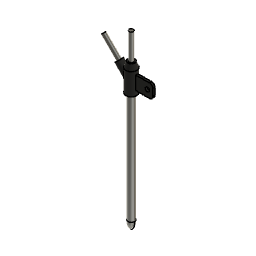
Pitot Tube Holybro (Autodesk Fusion 360 design; units mm, degrees)
Autodesk Fusion 360 part; units mm, degrees
sketch "Sketch1" plane through (0, 0, 0) normal (0, 0, 1) x (1, 0, 0)
  circle A0 centre (0, 0) radius 3.25
  dimension "d1" = 6.5
  constraint coincident A0.centre origin
  measures "d1" diameter of A0
extrude "Extrude1" add sketch "Sketch1" along normal blind 13 makes body 1
ref_plane "WorkPlane1" through (0, 0, 16.3) normal (0, 0, 1) x (1, 0, 0)
sketch "Sketch2" plane through (0, 0, 16.3) normal (0, 0, 1) x (1, 0, 0)
  circle A0 centre (0, 0) radius 2.15
  dimension "d5" = 4.3
  constraint coincident A0.centre origin
  measures "d5" diameter of A0
loft "Loft1" add profiles "Sketch2" section 1 face at (0.0595, 0.9382, 13) section 2 on bodies 1 bodies 1
sketch "Sketch3" plane through (0, 0, 16.3) normal (0, 0, 1) x (-1, 0, 0)
  circle A0 centre (0, 0) radius 2.15
  circle A1 centre (0, 0) radius 1.25
  dimension "d6" = 2.5
  constraint concentric A0 A1
  measures "d6" diameter of A1
extrude "Extrude2" add sketch "Sketch3" along normal blind 15.75 separate body contours A1 makes body 2
sketch "Sketch4" plane through (0, 0, 0) normal (0, 1, 0) x (1, 0, 0)
  line L0 (-3.25, -13) -> (3.25, -13)
  line L1 (-3.25, 0) -> (3.25, 0)
  line L2 (3.25, 0) -> (3.25, -13)
  line L3 (3.25, -3) -> (3.25, -11)
  line L4 (0, -3) -> (13.45, -3)
  line L5 (13.45, -3) -> (13.45, -11)
  line L6 (13.45, -11) -> (0, -11)
  line L7 (0, -11) -> (0, -3)
  circle A0 centre (10.25, -7) radius 1.25
  dimension "d12" = 10.2
  dimension "d13" = 3
  dimension "d14" = 8
  dimension "d15" = 4
  dimension "d16" = 3.2
  dimension "d17" = 2.5
  constraint coincident L1.end L2.start
  constraint coincident L0.end L2.end
  constraint vertical L3
  constraint coincident L2 L3.end
  constraint horizontal L4
  constraint vertical L5
  constraint horizontal L6
  constraint vertical L7
  constraint coincident origin L7
  measures "d12" distance of L1.end L5
  measures "d13" distance of L1.end L4
  measures "d14" distance of L4.end L5.end
  measures "d15" distance of L4 A0.centre
  measures "d16" distance of L5 A0.centre
  measures "d17" diameter of A0
extrude "Extrude3" add sketch "Sketch4" along normal mid plane 1.3 contours L2 L3 L4 L5 L6 bodies 2 1
fillet "Fillet1" radius 1.85 2 edges at (13.45, 0, 11) (13.45, 0, 3) on bodies 1
sketch "Sketch5" plane through (0, 0, 0) normal (0, 0, -1) x (1, 0, 0)
  circle A0 centre (0, 0) radius 3.25
  circle A1 centre (0, 0) radius 2
  dimension "d22" = 4
  constraint coincident A0.centre A1.centre
  measures "d22" diameter of A1
extrude "Extrude4" add sketch "Sketch5" along normal blind 65.7 separate body contours A1 makes body 3
sketch "Sketch6" plane through (0, 0, 0) normal (0, 1, 0) x (1, 0, 0)
  line L0 (2, 65.7) -> (-2, 65.7)
  line L1 (0, 65.7) -> (0, 70.7)
  line L2 (0, 70.7) -> (0.2, 70.7)
  spline S0 degree 5 poles (2, 65.7) (2, 65.822) (1.9982, 66.0643) (1.9904, 66.4231) (1.9681, 66.8915) (1.9135, 67.4579) (1.8222, 68.0018) (1.6848, 68.5199) (1.4938, 69.0096) (1.2482, 69.4714) (0.9504, 69.9067) (0.6731, 70.2355) (0.4445, 70.4717) (0.283, 70.6246) (0.2, 70.7) knots 0 0 0 0 0 0 0.1 0.2 0.3 0.4 0.5 0.6 0.7 0.8 0.9 1 1 1 1 1 1
  line L3 (2, 65.0687) -> (2, 66.3313)
  line L4 (2, 65.7) -> (0, 65.7)
  point P0 (1.6554, 68.5611)
  dimension "d25" = 5
  dimension "d26" = 0.2
  constraint midpoint L0 L1.start
  constraint perpendicular L0 L1
  constraint perpendicular L1 L2
  constraint coincident L0.start S0.start
  constraint midpoint L0.start L3
  constraint vertical L3
  measures "d25" distance of L1.start L1.end
  measures "d26" distance of L1.end L2.end
revolve "Revolve1" add sketch "Sketch6" angle 360 about axis through (0, 0, -65.7) along (0, 0, -1) bodies 3
ref_plane "WorkPlane2" through (0, 12.125, 0) normal (-0.707107, 0, 0.707107) x (0, 1, 0)
sketch "Sketch7" plane through (0, 12.125, 0) normal (-0.707107, 0, 0.707107) x (0, 1, 0)
sketch "Sketch8" plane through (0, 12.125, 0) normal (-0.707107, 0, 0.707107) x (0, 1, 0)
  line L0 (-12.125, -1.2374) -> (-12.125, -15.9099)
  circle A0 centre (-12.125, -4.3) radius 1.25
  circle A1 centre (-12.125, -4.3) radius 2.3
  point P0 (-12.125, 0)
  dimension "d29" = 4.3
  dimension "d30" = 2.5
  dimension "d34" = 4.6
  constraint coincident L0 A0.centre
  constraint concentric A0 A1
  measures "d29" distance of P0 A0.centre
  measures "d30" diameter of A0
  measures "d34" diameter of A1
extrude "Extrude6" add sketch "Sketch8" along normal blind 9.4 from surface at 5 bodies 1
extrude "Extrude5" add sketch "Sketch8" along normal blind 21.6 from surface at 6 separate body contours L0 A0 | L0 A0 makes body 4
